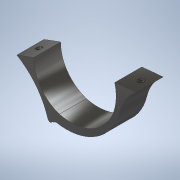
# Autodesk Inventor part: Part47
Saved by Autodesk Inventor 2021 (Build 250183000, 183)
## iProperties
Created: 2020-11-22
Part Number: Part47
Material: Liga de Nickel-Copper 400
Document SubType Name: Modeling
Designer: Lucas Moura
Density: 8.83 g/cm^3
Appearance: Cromado - Preto polido
Author: Lucas Moura
Autodesk Inventor part; units mm, degrees
ref_plane "YZ Plane" through (0, 0, 0) normal (1, 0, 0) x (0, 1, 0)
sketch "Sketch1" plane through (0, 0, 0) normal (0, 0, 1) x (1, 0, 0)
  arc A0 (10.3242, -27.9992) -> (11.7654, -28.1173) centre (11.0677, -27.7785) ccw
  line L0 (11.7654, -28.1173) -> (12.9919, -27.5665)
  arc A1 (12.9919, -27.5665) -> (34.2886, -13.9193) centre (16.4917, -9.5875) ccw
  arc A2 (10.3242, -27.9992) -> (0, -14.7343) centre (-11.7995, -34.5682) ccw
  arc A3 (5.5815, -12.6488) -> (14.136, -24.6939) centre (18.1207, -12.8036) ccw
  arc A4 (32.6339, -13.5274) -> (32.5628, -6.3713) centre (17.9412, -10.0948) ccw
  arc A5 (39.6875, -5.6924) -> (34.2886, -13.9193) centre (48.5431, -17.3889) ccw
  arc A6 (5.5815, -12.6488) -> (0, -14.7343) centre (48.5171, -136.0683) ccw
  arc A7 (39.6875, -5.6924) -> (32.5628, -6.3713) centre (48.5171, -136.0683) ccw
  arc A8 (14.136, -24.6939) -> (32.6339, -13.5274) centre (17.9429, -10.0956) ccw
  point P0 (0, 0)
  constraints: 18 point on circle, 9 centre point, 2 end point, 2 tangent
extrude "Extrusion1" add sketch "Sketch1" along normal blind 8.98
ref_plane "Work Plane1" through (39.6875, -5.6924, 0) normal (-0.0676, 0.9977, 0) x (-0.9977, -0.0676, 0)
sketch "Sketch2" plane through (39.6875, -5.6924, 0) normal (-0.0676, 0.9977, 0) x (-0.9977, -0.0676, 0)
  circle A0 centre (2.81, 4.525) radius 1
  line L0 (7.1542, 0) -> (0, 0) projected
  line L1 (0, 0) -> (0, 8.98) projected
  point P0 (39.2122, 0)
  dimension "d2" = 2
  dimension "d15" = 4.525
  dimension "d16" = 2.81
  constraints: 1 centre point
  measures "d2" diameter of A0
  measures "d15" distance from line of L0 A0.centre
  measures "d16" distance from line of L1 A0.centre
extrude "Extrusion2" cut sketch "Sketch2" against normal through all
thread "Thread1" size "M2x0.4" class "6H" standard "ANSI Metric M Profile" full length
ref_plane "Work Plane2" through (0, -14.7343, 0) normal (-0.3713, 0.9285, 0) x (-0.9285, -0.3713, 0)
sketch "Sketch3" plane through (0, -14.7343, 0) normal (-0.3713, 0.9285, 0) x (-0.9285, -0.3713, 0)
  circle A0 centre (-3, 4.455) radius 1
  line L0 (0, 0) -> (0, 8.98) projected
  line L1 (0, 8.98) -> (-5.9568, 8.98) projected
  line L2 (0, 0) -> (-5.9568, 0) projected
  point P0 (-5.4706, 0)
  dimension "d7" = 2
  dimension "d12" = 3
  dimension "d13" = 4.525
  dimension "d14" = 8.98
  constraints: 1 centre point
  measures "d7" diameter of A0
  measures "d12" distance from line of A0.centre L0
  measures "d13" distance from line of L1 A0.centre
  measures "d14" distance between parallel lines of L1 L2
extrude "Extrusion3" cut sketch "Sketch3" against normal through all
thread "Thread2" size "M2x0.4" class "6H" standard "ANSI Metric M Profile" full length
body "Solid1"
